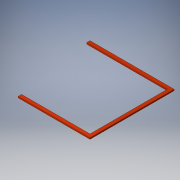
# Autodesk Inventor part: Base for Pool House
Saved by Autodesk Inventor 2016 (Build 200138000, 138)
## iProperties
Created: 2015-05-30
Part Number: Base for Pool House
Material: Wood (Oak)
Document SubType Name: Modeling
Designer: steele
Density: 0.76 g/cm^3
Appearance: White Oak - Natural Medium Gloss
Author: steele
Autodesk Inventor part; units mm, degrees
ref_plane "YZ Plane" through (0, 0, 0) normal (1, 0, 0) x (0, 1, 0)
ref_plane "XZ Plane" through (0, 0, 0) normal (0, 1, 0) x (-1, 0, 0)
ref_plane "XY Plane" through (0, 0, 0) normal (0, 0, 1) x (1, 0, 0)
sketch "Sketch1" plane through (0, 0, 0) normal (0, 1, 0) x (-1, 0, 0)
  line L0 (-44.45, 1130.3) -> (-44.45, -1130.3)
  line L1 (-44.45, -1130.3) -> (44.45, -1130.3)
  line L2 (44.45, -1041.4) -> (44.45, 1130.3)
  line L3 (44.45, 1130.3) -> (-44.45, 1130.3)
  line L4 (-44.45, 1130.3) -> (44.45, -1130.3) construction
  line L5 (-44.45, -1130.3) -> (44.45, 1130.3) construction
  line L6 (44.45, 1130.3) -> (1885.95, 1130.3)
  line L7 (1885.95, 1130.3) -> (1885.95, 1041.4)
  line L8 (1795.9397, 1041.4) -> (44.45, 1041.4)
  line L9 (44.45, 1041.4) -> (44.45, 1130.3)
  line L10 (44.45, -1130.3) -> (2216.15, -1130.3)
  line L11 (2216.15, -1130.3) -> (2216.15, -1041.4)
  line L12 (2126.1397, -1041.4) -> (44.45, -1041.4)
  line L13 (44.45, -1041.4) -> (44.45, -1130.3)
  line L14 (2128.3466, -1055.3201) -> (2126.1397, -1041.4) construction
  line L15 (1885.95, 1041.4) -> (1798.1466, 1027.4799) construction
  line L16 (2216.15, -1041.4) -> (2126.1397, -1041.4)
  line L17 (1885.95, 1041.4) -> (1795.9397, 1041.4)
  point P0 (0, 0)
  dimension "d0" = 88.9
  dimension "d1" = 2260.6
  dimension "d3" = 1930.4
  dimension "d5" = 2260.6
  dimension "d16" = 88.9
  dimension "d17" = 88.9
  constraints: 36 end point, 6 parallel, 4 horizontal, 3 perpendicular, 2 midpoint, 1 vertical
  measures "d0" distance of L1.end L0.end
  measures "d1" distance of L0.start L0.end
  measures "d3" distance between parallel lines of L7 L0
  measures "d5" distance between parallel lines of L11 L0
  measures "d16" distance between parallel lines of L10 L12
  measures "d17" distance between parallel lines of L8 L6
extrude "Extrusion1" add sketch "Sketch1" along normal blind 38.1
body "Solid1"
